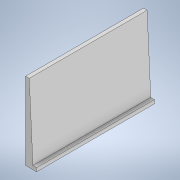
# Autodesk Inventor part: TurretBracket
Saved by Autodesk Inventor 2022 (Build 260153000, 153)
## iProperties
Created: 2022-03-03
Part Number: TurretBracket
Material: Generic
Document SubType Name: Modeling
Designer: merky
Density: 1 g/cm^3
Appearance: Default
Author: merky
Autodesk Inventor part; units mm, degrees
ref_plane "YZ Plane" through (0, 0, 0) normal (1, 0, 0) x (0, 1, 0)
ref_plane "XZ Plane" through (0, 0, 0) normal (0, 1, 0) x (-1, 0, 0)
ref_plane "XY Plane" through (0, 0, 0) normal (0, 0, 1) x (1, 0, 0)
sketch "Sketch1" plane through (0, 0, 0) normal (0, 0, 1) x (1, 0, 0)
  line L0 (0, 0) -> (19.05, 0)
  line L1 (19.05, 0) -> (19.05, 6.35)
  line L2 (19.05, 6.35) -> (0, 6.35)
  line L3 (0, 6.35) -> (0, 0)
  line L4 (0, 6.35) -> (6.35, 6.35)
  line L5 (6.35, 6.35) -> (6.35, 133.35)
  line L6 (6.35, 133.35) -> (0, 133.35)
  line L7 (0, 133.35) -> (0, 6.35)
  line L8 (12.7, 6.35) -> (6.35, 133.35)
  dimension "d0" = 19.05
  dimension "d1" = 6.35
  dimension "d2" = 6.35
  dimension "d3" = 127
  constraints: 18 end point, 4 parallel, 2 horizontal, 2 perpendicular, 1 point on line
  measures "d0" distance of L2.end L1.end
  measures "d1" distance of L1.end L0.end
  measures "d2" distance of L6.end L5.end
  measures "d3" distance of L5.end L4.end
extrude "Extrusion1" add sketch "Sketch1" along normal blind 203.2
body "Solid1"
